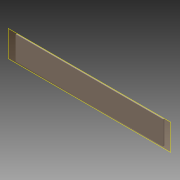
# Autodesk Inventor part: Panel_front
Saved by Autodesk Inventor 2013 (Build 170138000, 138)
## iProperties
Created: 2013-02-02
Part Number: Panel_front
Material: Aluminum 6061
Document SubType Name: Modeling
Designer: xylzlyx
Density: 1 g/cm^3
Author: xylzlyx
Autodesk Inventor part; units mm, degrees
ref_plane "YZ Plane" through (0, 0, 0) normal (1, 0, 0) x (0, 1, 0)
ref_plane "XZ Plane" through (0, 0, 0) normal (0, 1, 0) x (-1, 0, 0)
ref_plane "XY Plane" through (0, 0, 0) normal (0, 0, 1) x (1, 0, 0)
ref_plane "Work Plane1" through (0, 0, -12.7) normal (0, 0, 1) x (1, 0, 0)
sketch "Sketch1" plane through (0, 0, -12.7) normal (0, 0, 1) x (1, 0, 0)
  line L0 (381, -61.3641) -> (381, -64.5881) construction
  line L1 (381, -64.5881) -> (0, -64.5881) construction
  line L2 (0, -64.5881) -> (0, -61.3641) construction
  line L3 (0, -61.3641) -> (381, -61.3641) construction
  line L4 (381, 0) -> (0, 0) construction
  line L5 (0, 0) -> (0, 3.175) construction
  line L6 (0, 3.175) -> (381, 3.175) construction
  line L7 (381, 3.175) -> (381, 0) construction
  line L8 (381, -61.3641) -> (0, -61.3641)
  line L9 (0, -61.3641) -> (0, 0)
  line L10 (0, 0) -> (381, 0)
  line L11 (381, 0) -> (381, -61.3641)
  constraints: 24 end point, 5 horizontal, 4 coincident, 4 vertical, 2 parallel, 1 perpendicular, 7 other
extrude "FrontPanel" add sketch "Sketch1" against normal blind 3.175
fillet "Fillet1" radius 1 4 edges at (381, -61.3641, -14.2875) (381, 0, -14.2875) (0, -61.3641, -14.2875) (0, 0, -14.2875)
body "Solid1"
